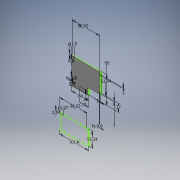
# Autodesk Inventor part: support arduino
Saved by Autodesk Inventor 2016 (Build 200138000, 138)
## iProperties
Created: 2018-04-23
Part Number: support arduino
Material: Generic
Document SubType Name: Modeling
Designer: mbouhier
Density: 1 g/cm^3
Appearance: Default
Author: mbouhier
Autodesk Inventor part; units mm, degrees
ref_plane "YZ Plane" through (0, 0, 0) normal (1, 0, 0) x (0, 1, 0)
ref_plane "XZ Plane" through (0, 0, 0) normal (0, 1, 0) x (-1, 0, 0)
ref_plane "XY Plane" through (0, 0, 0) normal (0, 0, 1) x (1, 0, 0)
sketch "Sketch1" plane through (0, 0, 0) normal (0, 1, 0) x (-1, 0, 0)
  line L0 (-49.1271, 39.6605) -> (50.3929, 39.6605)
  line L1 (50.3929, 39.6605) -> (50.3929, -31.3395)
  line L2 (25.123, -55.3395) -> (-6.6071, -55.3395)
  line L3 (95, -161) -> (-6.6, -161)
  line L4 (-6.6, -161) -> (-6.6, -214.34)
  line L5 (-6.6, -214.34) -> (95, -214.34)
  line L6 (95, -214.34) -> (95, -161)
  line L7 (-46.1271, 25.2005) -> (-46.1271, -28.3395)
  line L8 (-46.1271, -28.3395) -> (50.3929, -28.3395)
  line L9 (-49.1271, 28.2005) -> (-49.1271, -31.3395)
  line L10 (50.3929, -31.3395) -> (-49.1271, -31.3395)
  line L11 (-46.1271, 25.2005) -> (50.3929, 25.2005)
  line L12 (-46.1271, 28.2005) -> (50.3929, 28.2005)
  line L13 (-46.1271, 28.2005) -> (-49.1271, 28.2005)
  line L14 (49.5929, 24.4005) -> (-45.3271, 24.4005)
  line L15 (-45.3271, 24.4005) -> (-45.3271, -27.5395)
  line L16 (-45.3271, -27.5395) -> (49.5929, -27.5395)
  line L17 (50.3929, -26.6821) -> (50.3929, 25.2579)
  line L18 (50.3929, 39.6605) -> (53.3929, 39.6605)
  line L19 (53.3929, 39.6605) -> (53.3929, -34.4821)
  line L20 (50.3929, -34.4821) -> (50.3929, 39.6605)
  line L21 (50.3929, 28.2005) -> (53.3929, 28.2005)
  line L22 (50.3929, -31.3395) -> (53.3929, -31.3395)
  line L23 (49.5929, 24.4005) -> (49.5929, -27.5395)
  line L24 (53.3929, -34.4821) -> (53.3929, -55.3395)
  line L25 (53.3929, -55.3395) -> (25.123, -55.3395)
  line L26 (-6.6071, -31.3395) -> (-6.6071, -55.3395)
  line L27 (-49.1271, 28.2005) -> (-49.1271, 39.6605)
  point P0 (-49.6071, -31.3395)
  point P1 (81.03, -163.54)
  point P2 (-1.52, -163.54)
  point P3 (-1.52, -163.54)
  point P4 (41.8929, 33.6605)
  point P5 (23.3929, -45.3395)
  dimension "d8" = 101.6
  dimension "d9" = 53.34
  dimension "d10" = 13.97
  dimension "d11" = 2.54
  dimension "d12" = 96.52
  dimension "d13" = 96.52
  dimension "d14" = 27
  dimension "d15" = 3
  dimension "d17" = 3
  dimension "d20" = 53.54
  dimension "d21" = 3
  dimension "d23" = 6
  dimension "d24" = 10
  dimension "d28" = 0.8
  dimension "d29" = 0.8
  dimension "d30" = 0.8
  dimension "d46" = 3
  dimension "d47" = 0.8
  dimension "d48" = 11.5
  dimension "d49" = 60
  dimension "d51" = 30
  dimension "d52" = 95
  constraints: 56 end point, 16 perpendicular, 8 point on line, 6 parallel, 4 horizontal, 2 vertical, 1 coincident
  measures "d8" distance of L5.end L4.end
  measures "d9" distance of L4.end L3.end
  measures "d10" distance from line of point (81.03, -163.54) L6
  measures "d11" distance from line of point (81.03, -163.54) L3
  measures "d12" distance from line of point (-1.52, -163.54) L6
  measures "d13" distance between parallel lines of L7 L1
  measures "d14" distance between parallel lines of L2 L8
  measures "d15" distance between parallel lines of L7 L9
  measures "d17" distance between parallel lines of L10 L8
  measures "d20" distance from line of L7.start L8
  measures "d21" distance between parallel lines of L12 L11
  measures "d23" distance from line of point (41.893, 33.66) L0
  measures "d24" distance from line of point (23.393, -45.34) L2
  measures "d28" distance between parallel lines of L14 L11
  measures "d29" distance between parallel lines of L7 L15
  measures "d30" distance between parallel lines of L8 L16
  measures "d46" distance of L19.end L20.start
  measures "d47" distance between parallel lines of L1 L23
  measures "d48" distance from line of point (41.893, 33.66) L19
  measures "d49" distance between parallel lines of L26 L24
  measures "d51" distance from line of point (23.393, -45.34) L26
  measures "d52" distance between parallel lines of L0 L25
extrude "Extrusion1" add sketch "Sketch1" against normal blind 3 contours L0 L1 L12 L13 L27 | L18 L19 L21 L1 | L13 L12 L1 L11 L7 L8 L10 L9 | L10 L22 L19 L24 L25 L2 L26 | L1 L8 L7 L11 | L23 L16 L15 L14
fillet "Fillet1" radius 5 1 edges at (49.1271, -1.5, 39.6605)
fillet "Fillet2" radius 3 1 edges at (-53.3929, -1.5, 39.6605)
extrude "Extrusion2" add sketch "Sketch1" along normal blind 5 contours L13 L12 L1 L11 L7 L8 L10 L9 | L21 L19 L22 L1
extrude "Extrusion3" add sketch "Sketch1" along normal blind 3 contours L1 L8 L7 L11
hole "Hole1" at (-81.03, 0, -163.54) at (1.52, 0, -163.54) at (-41.8929, 0, 33.6605) at (-23.3929, 0, -45.3395) direction (0, -1, 0) diameter 4.5 end through all
fillet "Fillet3" radius 5 1 edges at (6.6071, -1.5, -31.3395)
equation "\"d29\" = d28"
equation "\"d30\" = d28"
body "Solid1"
